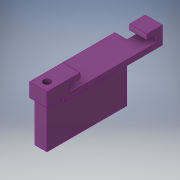
# Autodesk Inventor part: 000.702 - Активный прижим
Saved by Autodesk Inventor 2019 (Build 230136000, 136)
## iProperties
Created: 2020-02-29
Part Number: 000.702 - Активный прижим
Material: Пластик АБС
Document SubType Name: Modeling
Designer: Петров Иван
Density: 1.06 g/cm^3
Appearance: Гладкий — пурпурный
Author: Петров Иван
Autodesk Inventor part; units mm, degrees
ref_plane "YZ Plane" through (0, 0, 0) normal (1, 0, 0) x (0, 1, 0)
ref_plane "XZ Plane" through (0, 0, 0) normal (0, 1, 0) x (-1, 0, 0)
ref_plane "XY Plane" through (0, 0, 0) normal (0, 0, 1) x (1, 0, 0)
sketch "Эскиз1" plane through (0, 0, 0) normal (1, 0, 0) x (0, 1, 0)
  line L0 (-2, 25.25) -> (2, 25.25)
  line L1 (2, 25.25) -> (2, -25.25)
  line L2 (2, -25.25) -> (-2, -25.25)
  line L3 (-2, -25.25) -> (-2, 25.25)
  line L4 (-2, 25.25) -> (2, -25.25) construction
  line L5 (2, 25.25) -> (-2, -25.25) construction
  line L6 (2, 25.25) -> (5, 25.25)
  line L7 (5, 25.25) -> (5, 19.25)
  line L8 (5, 19.25) -> (2, 19.25)
  line L9 (2, 19.25) -> (2, 25.25)
  line L10 (2, -25.25) -> (5, -25.25)
  line L11 (5, -25.25) -> (5, -19.25)
  line L12 (5, -19.25) -> (2, -19.25)
  line L13 (2, -19.25) -> (2, -25.25)
  line L14 (5, 25.25) -> (-5, 25.25)
  line L15 (-5, 25.25) -> (-5, 28.25)
  line L16 (-5, 28.25) -> (5, 28.25)
  line L17 (5, 28.25) -> (5, 25.25)
  line L18 (5, -25.25) -> (-5, -25.25)
  line L19 (-5, -25.25) -> (-5, -28.25)
  line L20 (-5, -28.25) -> (5, -28.25)
  line L21 (5, -28.25) -> (5, -25.25)
  line L22 (-5, 28.25) -> (-2, 28.25)
  line L23 (-2, 28.25) -> (-2, -28.25)
  line L24 (-2, -28.25) -> (-5, -28.25)
  line L25 (-5, -28.25) -> (-5, 28.25)
  point P0 (0, 0)
  dimension "d0" = 4
  dimension "d1" = 50.5
  dimension "d2" = 3
  dimension "d3" = 6
  dimension "d4" = 3
  dimension "d5" = 6
  dimension "d6" = 10
  dimension "d7" = 10
  dimension "d8" = 3
  dimension "d9" = 3
  constraints: 52 end point, 12 parallel, 6 horizontal, 6 perpendicular, 2 midpoint, 2 point on line
  measures "d0" distance of L1.end L2.end
  measures "d1" distance of L0.end L1.end
  measures "d2" distance of L7.end L8.end
  measures "d3" distance of L6.end L7.end
  measures "d4" distance of L12.end L11.end
  measures "d5" distance of L11.end L10.end
  measures "d6" distance of L15.end L16.end
  measures "d7" distance of L20.end L19.end
  measures "d8" distance of L19.end L18.end
  measures "d9" distance of L16.end L6.end
extrude "Выдавливание1" add sketch "Эскиз1" along normal blind 10 contours L23 L16 L17 L6 L0 | L3 L18 L25 L14 | L14 L15 L16 L23 | L6 L7 L8 L1 | L23 L20 L19 L18 | L2 L10 L21 L20 L23 | L1 L12 L11 L10
sketch "Эскиз2" plane through (0, -5, -28.25) normal (0, -1, 0) x (1, 0, 0)
  line L0 (10, 47.5) -> (10, 56.5) projected
  line L1 (10, 56.5) -> (0, 56.5)
  line L2 (0, 56.5) -> (0, 66.5)
  line L3 (0, 66.5) -> (10, 66.5)
  line L4 (10, 66.5) -> (10, 56.5)
  circle A0 centre (5, 61.5) radius 2
  line L5 (0, 61.5) -> (3, 61.5)
  line L6 (7, 61.5) -> (10, 61.5)
  point P0 (0, 28.25)
  dimension "d14" = 10
  dimension "d15" = 10
  dimension "d29" = 4
  dimension "d30" = 5
  dimension "d31" = 5
  constraints: 12 end point, 2 midpoint, 2 parallel, 2 point on circle, 1 centre point, 1 horizontal, 1 perpendicular
  measures "d14" distance of L2.end L3.end
  measures "d15" distance of L1.end L2.end
  measures "d29" diameter of A0
  measures "d30" distance from line of L2 A0.centre
  measures "d31" distance from line of L3 A0.centre
extrude "Выдавливание2" add sketch "Эскиз2" against normal blind 10 contours L1 L2 L5 A0 L6 L4 | L6 A0 L5 L2 L3 L4
sketch "Эскиз3" plane through (0, -5, -28.25) normal (0, -1, 0) x (1, 0, 0)
  line L0 (0, 56.5) -> (10, 56.5) projected
  line L1 (0, 56.5) -> (-7, 56.5)
  line L2 (-7, 56.5) -> (-7, 10.5)
  line L3 (-7, 10.5) -> (0, 10.5)
  line L4 (0, 10.5) -> (0, 56.5)
  point P0 (0, 28.25)
  dimension "d21" = 7
  constraints: 8 end point, 2 parallel, 1 horizontal, 1 perpendicular
  measures "d21" distance of L3.end L2.end
extrude "Выдавливание3" add sketch "Эскиз3" along normal blind 30 and the other way blind 1
sketch "Эскиз4" plane through (0, -5, -28.25) normal (0, -1, 0) x (1, 0, 0)
  line L0 (10, 47.5) -> (10, 56.5)
  line L1 (10, 56.5) -> (0, 56.5)
  line L2 (0, 56.5) -> (0, 66.5)
  line L3 (0, 66.5) -> (10, 66.5)
  line L4 (10, 66.5) -> (10, 56.5)
  circle A0 centre (5, 61.5) radius 2
  line L5 (0, 61.5) -> (3, 61.5)
  line L6 (7, 61.5) -> (10, 61.5)
  point P0 (0, 28.25)
  point P1 (0, 28.25)
  dimension "d32" = 10
  dimension "d33" = 10
  dimension "d34" = 4
  dimension "d35" = 5
  dimension "d36" = 5
  constraints: 14 end point, 2 midpoint, 2 parallel, 2 point on circle, 1 centre point, 1 horizontal, 1 perpendicular
  measures "d32" distance of L2.end L3.end
  measures "d33" distance of L1.end L2.end
  measures "d34" diameter of A0
  measures "d35" distance from line of L2 A0.centre
  measures "d36" distance from line of L3 A0.centre
extrude "Выдавливание4" cut sketch "Эскиз4" against normal blind 2 contours L1 L2 L5 A0 L6 L4 | L6 A0 L5 L2 L3 L4
move faces "Перенос1" translate (0, 2, 0) faces at (-2.3333, -4, -2.4167) (0, -15, -2.4167)
